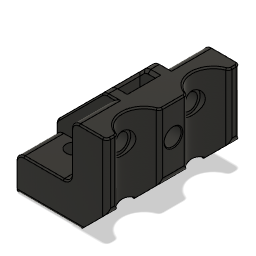
Apollo Yoke Int. Corner P2 [(P)MPLA000000157] v1 (Autodesk Fusion 360 design; units mm, degrees)
Autodesk Fusion 360 part; units mm, degrees
note: some values were not read from the file. Chosen so that the rebuilt part matches the saved one: which face or edge a step refers to; which pieces of a blend or face edit are solid. Set by a fixed rule: which sketch regions a step uses.
sketch "Sketch1" plane through (0, 0, 0) normal (0, 1, 0) x (1, 0, 0)
  line L0 (-17, 25) -> (-17, -25)
  line L1 (17, 25) -> (17, -25)
  line L2 (-17, -25) -> (17, -25)
  circle A0 centre (-19, 13) radius 8.1
  circle A1 centre (-19, -13) radius 8.1
  line L3 (-17, 25) -> (17, 25)
  circle A2 centre (19, 13) radius 8.1
  circle A3 centre (19, -13) radius 8.1
  dimension "d7" = 50
  dimension "d8" = 25
  dimension "d74" = 16.2
  dimension "d75" = 16.2
  dimension "d97" = 34
  dimension "d100" = 17
  dimension "d101" = 16.2
  dimension "d102" = 16.2
  dimension "d103" = 38
  dimension "d104" = 26
  dimension "d105" = 13
  dimension "d106" = 19
  constraint vertical L0
  constraint vertical L1
  constraint horizontal L2
  constraint horizontal L3
  constraint vertical A3.centre A2.centre
  constraint horizontal A0.centre A2.centre
  constraint horizontal A1.centre A3.centre
  constraint vertical A0.centre A1.centre
  measures "d7" distance of L2 L3
  measures "d8" distance of origin L2
  measures "d74" diameter of A3
  measures "d75" diameter of A2
  measures "d97" distance of L0 L1
  measures "d100" distance of origin L1
  measures "d101" diameter of A0
  measures "d102" diameter of A1
  measures "d103" distance of A0.centre A2.centre
  measures "d104" distance of A0.centre A1.centre
  measures "d105" vertical distance of origin A0.centre
  measures "d106" horizontal distance of origin A0.centre
extrude "Extrude1" add sketch "Sketch1" along normal blind 34 contours L0 L1 L2 A0 A1 L3 A2 A3 | L0 A0 | L0 A1 picked at (-15.419, 11.504) picked at (-14.0304, -14.3154)
sketch "Sketch3" plane through (17, 0, 0) normal (1, 0, 0) x (0, 0, -1)
  line L0 (20.8492, 0) -> (25, 0)
  line L1 (25, 0) -> (25, 34)
  line L2 (25, 34) -> (20.8492, 34)
  line L3 (-25, 34) -> (-25, 0)
  circle A0 centre (-13, -2) radius 8
  circle A1 centre (13, -2) radius 8.2
  circle A2 centre (-13, -2) radius 8.2
  circle A3 centre (13, -2) radius 8
  line L4 (20.8492, 34) -> (20.8492, 0)
  line L5 (-25, 0) -> (-20.8492, 0)
  line L6 (-20.8492, 0) -> (-20.8492, 34)
  line L7 (-20.8492, 34) -> (-25, 34)
  dimension "d34" = 0.2
  dimension "d35" = 0.2
  dimension "d36" = 16
  dimension "d37" = 16
  dimension "d38" = 26
  dimension "d39" = 13
  dimension "d40" = 2
  constraint concentric A0 A2
  constraint concentric A1 A3
  constraint horizontal A0.centre A1.centre
  measures "d36" diameter of A0
  measures "d37" diameter of A3
  measures "d38" distance of A0.centre A1.centre
  measures "d39" horizontal distance of origin A0.centre
  measures "d40" vertical distance of origin A0.centre
extrude "Extrude4" cut sketch "Sketch3" against normal blind 34 contours A0 | A3
chamfer "Chamfer4" distance 10 angle 45 7 edges at (17, 0, -22.9246) (17, 0, 22.9246) (17, 0, -22.9246) (17, 0, 0) (17, 0, 22.9246) (17, 0, 0) (17, 0, -22.9246)
chamfer "Chamfer5" distance 18 angle 45 1 edges at (-17, 34, 0)
fillet "Fillet3" radius 1.5 12 edges at (-5, 0, -25) (-5, 0, 25) (-5, 0, 5.254) (-5, 0, 20.746) (-5, 0, -5.254) (-5, 0, -20.746) (17, 22, 20.8492) (17, 22, 5.1508) (17, 22, -5.1508) (17, 22, -20.8492) (17, 22, -25) (17, 22, 25)
fillet "Fillet4" radius 3 8 edges at (7, 0, -22.6659) (17, 10, -22.7196) (17, 10, 0) (7, 0, 0) (7, 0, 22.6659) (17, 10, 22.7196) (-17, 16, 0) (1, 34, 0)
chamfer "Chamfer3" distance 0.5 angle 45 41 edges at (8.8713, 34, -25) (1.0946, 33.7716, -25) (-8, 25, -25) (-16.7716, 15.9054, -25) (-17, 8.1287, -25) (-17, 0.4393, -24.5607) (-17, 0, -22.6659) (-17, 0.2592, -20.9888) (-17, 6, -13) (-17, 0.2592, -5.0112) (-17, 0, 0) (-17, 0, 22.6659) (-17, 0, -22.6659) (-17, 0.2592, 20.9888) (-17, 0.2592, 5.0112) (-17, 6, 13) (-17, 0.2592, 20.9888) (-17, 0, 22.6659) (-17, 0.4393, 24.5607) (-17, 8.1287, 25) (-16.7716, 15.9054, 25) (-8, 25, 25) (1.0946, 33.7716, 25) (8.8713, 34, 25) (16.5607, 34, 24.5607) (17, 34, 22.7196) (16.739, 34, 21.0938) (10.9, 34, 13) (16.739, 34, 21.0938) (16.739, 34, 4.9062) (17, 34, -22.7196) (17, 34, 22.7196) (17, 34, 0) (16.739, 34, -4.9062) (10.9, 34, -13) (16.739, 34, -4.9062) (16.739, 34, -21.0938) (17, 34, 0) (17, 34, -22.7196) (17, 34, 22.7196) (16.5607, 34, -24.5607)
sketch "Sketch2" plane through (17, 0, 0) normal (1, 0, 0) x (0, 0, -1)
  circle A0 centre (0, 22.5) radius 3.1
  circle A1 centre (0, 22.5) radius 5.5
  line L0 (4.0608, 33.5) -> (-4.0608, 33.5)
  line L1 (-4.0608, 33.5) -> (-4.0608, 11.2426)
  line L2 (-4.0608, 11.2426) -> (4.0608, 11.2426)
  line L3 (4.0608, 11.2426) -> (4.0608, 33.5)
  line L4 (-4.9919, 34) -> (-21.0081, 34)
  dimension "d15" = 6.2
  dimension "d17" = 11
  dimension "d107" = 11.5
  constraint vertical origin A0.centre
  constraint concentric A0 A1
  measures "d15" diameter of A0
  measures "d17" diameter of A1
  measures "d107" distance of A0.centre L4
hole "Hole1" at (17, 22.5, 0) direction (-1, 0, 0) diameter 6.4 depth 21 tip angle 118 countersink diameter 7 countersink angle 90
sketch "Sketch4" plane through (0, 0, 0) normal (0, -1, 0) x (1, 0, 0)
  circle A0 centre (-5.5, 0) radius 3
  line L0 (-5.5, 4.1682) -> (-5.5, -4.1682)
  line L1 (5.259, -23.5) -> (5.259, -21.8318)
  line L2 (5.259, -21.8318) -> (-5.259, -21.8318)
  line L3 (-5.259, -21.8318) -> (-5.259, -23.5)
  line L4 (-5.259, -23.5) -> (5.259, -23.5)
  line L5 (5.7574, -4.1682) -> (5.7574, 4.1682)
  line L6 (5.7574, 4.1682) -> (-16.5, 4.1682)
  line L7 (-16.5, -4.1682) -> (5.7574, -4.1682)
  line L8 (-16.5, 4.1682) -> (-16.5, -4.1682)
  line L9 (-17, 4.1682) -> (-17, -4.1682)
  dimension "d66" = 6
  dimension "d110" = 11.5
  constraint horizontal origin A0.centre
  constraint midpoint A0.centre L0
  measures "d66" diameter of A0
  measures "d110" distance of A0.centre L9
hole "Hole2" at (-5.5, 0, 0) direction (0, 1, 0) diameter 6.4 depth 21 tip angle 118 countersink diameter 7 countersink angle 90
sketch "Sketch6" plane through (0, 34, 0) normal (0, 1, 0) x (-1, 0, 0)
  line L0 (-2.2426, 24.5) -> (-15.5, 24.5)
  arc A0 (-15.5, 24.5) -> (-16.5, 23.5) centre (-15.5, 23.5) ccw
  line L1 (-16.5, 23.5) -> (-16.5, 21.9392)
  arc A1 (-16.5, 21.9392) -> (-15.8646, 21.0081) centre (-15.5, 21.9392) ccw
  arc A2 (-15.8646, 4.9919) -> (-15.8646, 21.0081) centre (-19, 13) ccw
  arc A3 (-15.8646, 4.9919) -> (-16.5, 4.0608) centre (-15.5, 4.0608) ccw
  line L2 (-16.5, 4.0608) -> (-16.5, -4.0608)
  arc A4 (-16.5, -4.0608) -> (-15.8646, -4.9919) centre (-15.5, -4.0608) ccw
  arc A5 (-15.8646, -21.0081) -> (-15.8646, -4.9919) centre (-19, -13) ccw
  arc A6 (-15.8646, -21.0081) -> (-16.5, -21.9392) centre (-15.5, -21.9392) ccw
  line L3 (-16.5, -21.9392) -> (-16.5, -23.5)
  arc A7 (-16.5, -23.5) -> (-15.5, -24.5) centre (-15.5, -23.5) ccw
  line L4 (-15.5, -24.5) -> (-2.2426, -24.5)
  line L5 (-2.2426, -24.5) -> (-2.2426, 24.5)
  line L6 (-17, 4.0608) -> (-17, -4.0608)
  line L7 (-5, -5.25) -> (0.8, -5.25)
  line L8 (0.8, -5.25) -> (0.8, 5.25)
  line L9 (0.8, 5.25) -> (-5, 5.25)
  line L10 (-5, 5.25) -> (-5, -5.25)
  line L11 (-5, -5.25) -> (0.8, 5.25) construction
  line L12 (0.8, -5.25) -> (-5, 5.25) construction
  point P0 (-2.1, 0)
  dimension "d144" = 5.8
  dimension "d145" = 10.5
  dimension "d146" = 5.25
  dimension "d149" = 12
  constraint horizontal L7
  constraint perpendicular L7 L8
  constraint parallel L7 L9
  constraint parallel L8 L10
  constraint coincident L11 P0
  constraint coincident L12 P0
  measures "d144" distance of L8 L10
  measures "d145" distance of L7 L9
  measures "d146" distance of origin L7
  measures "d149" distance of L6 L10
extrude "Extrude5" cut sketch "Sketch6" against normal blind 13 contours L5 L7 L8 L9 | L5 L7 L9 L10
sketch "Sketch8" plane through (5, 0, 0) normal (-1, 0, 0) x (0, 0, 1)
  arc A0 (2.8267, 21) -> (-2.8267, 21) centre (0, 22.5) ccw
  line L0 (2.8267, 21) -> (5.25, 21)
  line L1 (5.25, 21) -> (5.25, 34)
  line L2 (5.25, 34) -> (-5.25, 34)
  line L3 (-5.25, 34) -> (-5.25, 21)
  line L4 (-5.25, 21) -> (-2.8267, 21)
  line L5 (5.25, 25.0311) -> (0, 28.0622)
  line L6 (0, 28.0622) -> (-5.25, 25.0311)
  line L7 (-5.25, 25.0311) -> (-5.25, 18.9689)
  line L8 (-5.25, 18.9689) -> (0, 15.9378)
  line L9 (0, 15.9378) -> (5.25, 18.9689)
  line L10 (5.25, 18.9689) -> (5.25, 25.0311)
  point P0 (0, 22)
  dimension "d156" = 0.5
  constraint collinear L3 L7
  constraint vertical A0.centre P0
  measures "d156" distance of A0.centre P0
extrude "Extrude7" cut sketch "Sketch8" along normal up to surface (5.8 mm away) contours A0 L0 L4 L7 L8 L9 L10
sketch "Sketch7" plane through (-17, 0, 0) normal (-1, 0, 0) x (0, 0, 1)
  line L0 (24.5, 1.5) -> (24.5, 14.7574)
  line L1 (24.5, 14.7574) -> (-24.5, 14.7574)
  line L2 (-24.5, 14.7574) -> (-24.5, 1.5)
  arc A0 (-24.5, 1.5) -> (-23.5, 0.5) centre (-23.5, 1.5) ccw
  line L3 (-23.5, 0.5) -> (-21.8318, 0.5)
  arc A1 (-21.8318, 0.5) -> (-20.9021, 1.1316) centre (-21.8318, 1.5) ccw
  arc A2 (-5.0979, 1.1316) -> (-20.9021, 1.1316) centre (-13, -2) ccw
  arc A3 (-5.0979, 1.1316) -> (-4.1682, 0.5) centre (-4.1682, 1.5) ccw
  line L4 (-4.1682, 0.5) -> (4.1682, 0.5)
  arc A4 (4.1682, 0.5) -> (5.0979, 1.1316) centre (4.1682, 1.5) ccw
  arc A5 (20.9021, 1.1316) -> (5.0979, 1.1316) centre (13, -2) ccw
  arc A6 (20.9021, 1.1316) -> (21.8318, 0.5) centre (21.8318, 1.5) ccw
  line L5 (21.8318, 0.5) -> (23.5, 0.5)
  arc A7 (23.5, 0.5) -> (24.5, 1.5) centre (23.5, 1.5) ccw
  line L6 (-4.1682, 0) -> (4.1682, 0)
  line L7 (5.25, 17.8) -> (-5.25, 17.8)
  line L8 (-5.25, 17.8) -> (-5.25, 12)
  line L9 (-5.25, 12) -> (5.25, 12)
  line L10 (5.25, 12) -> (5.25, 17.8)
  line L11 (5.25, 17.8) -> (-5.25, 12) construction
  line L12 (-5.25, 17.8) -> (5.25, 12) construction
  line L13 (-5.25, 32.2) -> (-5.25, 33.1213)
  point P0 (0, 14.9)
  dimension "d128" = 10.5
  dimension "d129" = 5.8
  dimension "d148" = 12
  constraint horizontal L7
  constraint perpendicular L7 L8
  constraint parallel L7 L9
  constraint parallel L8 L10
  constraint coincident L11 P0
  constraint coincident L12 P0
  constraint collinear L8 L13
  measures "d128" distance of L8.end L9.end
  measures "d129" distance of L7.end L8.end
  measures "d148" distance of origin L9
extrude "Extrude6" cut sketch "Sketch7" against normal blind 13 contours L1 L8 L9 L10 | L1 L7 L8 L10
sketch "Sketch9" plane through (0, 12, 0) normal (0, 1, 0) x (-1, 0, 0)
  line L0 (4, -2.8267) -> (4, -5.25)
  line L1 (4, -5.25) -> (17, -5.25)
  line L2 (17, -5.25) -> (17, 5.25)
  line L3 (17, 5.25) -> (4, 5.25)
  line L4 (4, 5.25) -> (4, 2.8267)
  arc A0 (4, -2.8267) -> (4, 2.8267) centre (5.5, 0) ccw
  line L5 (8.0311, -5.25) -> (11.0622, 0)
  line L6 (11.0622, 0) -> (8.0311, 5.25)
  line L7 (8.0311, 5.25) -> (1.9689, 5.25)
  line L8 (1.9689, 5.25) -> (-1.0622, 0)
  line L9 (-1.0622, 0) -> (1.9689, -5.25)
  line L10 (1.9689, -5.25) -> (8.0311, -5.25)
  point P0 (5.5, 0)
  point P1 (5.5, 0)
  point P2 (5, 0)
  dimension "d157" = 0.5
  constraint coincident P1 P0
  constraint collinear L1 L10
  constraint horizontal P1 P2
  measures "d157" distance of P1 P2
extrude "Extrude8" cut sketch "Sketch9" along normal up to surface (5.8 mm away) contours L0 L1 L3 L4 A0 L5 L6 L7 L10 | L0 L4 A0 L7 L8 L9 L10
chamfer "Chamfer8" distance 2 angle 45 1 edges at (-0.8, 17.8, 0)
chamfer "Chamfer6" distance 1 angle 45 14 edges at (-16.7716, 15.9054, 5.25) (-15.6607, 17.3393, 5.25) (-17, 13.3787, 5.25) (-16.7716, 15.9054, -5.25) (-17, 13.3787, -5.25) (-15.6607, 17.3393, -5.25) (3.6213, 34, 5.25) (1.0946, 33.7716, 5.25) (-0.3393, 32.6607, 5.25) (3.6213, 34, -5.25) (1.0946, 33.7716, -5.25) (-0.3393, 32.6607, -5.25) (5, 34, 0) (-17, 12, 0)
sketch "Sketch10" plane through (0, 0, 25) normal (0, 0, 1) x (1, 0, 0)
  line L0 (-16.5, 14.7574) -> (-16.5, 1.5)
  line L1 (-16.5, 1.5) -> (8.5, 1.5)
  line L2 (8.5, 1.5) -> (15.5, 8.5)
  line L3 (15.5, 8.5) -> (15.5, 33.5)
  line L4 (15.5, 33.5) -> (2.2426, 33.5)
  arc A0 (2.2426, 33.5) -> (0.4749, 32.7678) centre (2.2426, 31) ccw
  line L5 (0.4749, 32.7678) -> (-15.7678, 16.5251)
  arc A1 (-15.7678, 16.5251) -> (-16.5, 14.7574) centre (-14, 14.7574) ccw
  line L6 (3.7426, 13.2574) -> (-20.6124, 13.2574)
  line L7 (-20.6124, 13.2574) -> (-3.4252, 34.9761)
  line L8 (-3.4252, 34.9761) -> (3.7426, 34.9761)
  line L9 (3.7426, 13.2574) -> (3.7426, 34.9761)
  dimension "d134" = 1.5
  dimension "d135" = 1.5
  constraint perpendicular L0 L6
  constraint horizontal L8
  constraint vertical L9
  measures "d134" distance of L4.end L9
  measures "d135" distance of L0.start L6
extrude "Extrude9" cut sketch "Sketch10" against normal blind 15 contours L0 L4 A0 L5 A1 L6 L9 | L0 L4 A0 L5 A1 L6 L7 L8 L9
extrude "Extrude10" cut sketch "Sketch10" along normal blind 15 from surface at -50 contours L0 L4 A0 L5 A1 L6 L9 | L0 L4 A0 L5 A1 L6 L7 L8 L9
fillet "Fillet5" radius 3 6 edges at (3.7426, 34, 17.25) (-17, 13.2574, 17.25) (3.7426, 13.2574, 17.5) (-17, 13.2574, -17.25) (3.7426, 13.2574, -17.5) (3.7426, 34, -17.25)
chamfer "Chamfer7" distance 0.5 angle 45 20 edges at (3.7426, 23.6287, 25) (2.864, 14.136, 25) (-6.6287, 13.2574, 25) (-15.4186, 12.9007, 25) (4.0993, 32.4186, 25) (3.7426, 23.6287, -25) (4.0993, 32.4186, -25) (-15.4186, 12.9007, -25) (-6.6287, 13.2574, -25) (2.864, 14.136, -25) (-8, 25, -10) (-16.7716, 15.9054, -10) (-17, 12.5074, -10) (4.4926, 34, -10) (1.0946, 33.7716, -10) (-8, 25, 10) (1.0946, 33.7716, 10) (4.4926, 34, 10) (-17, 12.5074, 10) (-16.7716, 15.9054, 10)
chamfer "Chamfer10" distance 1.4 angle 45 2 edges at (-0.8, 32.2, 0) (-15.2, 17.8, 0)
sketch "Sketch11" plane through (0, 0, -5.25) normal (0, 0, 1) x (1, 0, 0)
  line L0 (-0.8, 19.8) -> (-1.6311, 18.9689)
  line L1 (-0.8, 25.6966) -> (-8.6966, 17.8)
  line L2 (-8.6966, 16.4221) -> (-2.5708, 16.4221)
  line L3 (-2.5708, 16.4221) -> (0.213, 19.206)
  line L4 (0.213, 19.206) -> (0.213, 25.6966)
  line L5 (0.213, 25.6966) -> (-0.8, 25.6966)
  line L6 (-8.6966, 17.8) -> (-8.6966, 16.4221)
  line L7 (-13.7858, 17.8) -> (-15.4142, 16.1716)
  arc A0 (-15.4142, 16.1716) -> (-16, 14.7574) centre (-14, 14.7574) ccw
  line L8 (-16, 14.7574) -> (-16, 12)
  line L9 (-16, 12) -> (-1.9689, 12)
  line L10 (-2.8, 17.8) -> (-13.7858, 17.8)
  line L11 (5.1492, 19.0162) -> (-1.9689, 12)
  line L12 (5.1492, 19.0162) -> (-0.8, 19.8)
  line L13 (-1.9689, 12) -> (-1.6311, 18.9689)
  line L14 (5, 33) -> (2.2426, 33)
  arc A1 (2.2426, 33) -> (0.8284, 32.4142) centre (2.2426, 31) ccw
  line L15 (0.8284, 32.4142) -> (-0.8, 30.7858)
  line L16 (-0.8, 30.7858) -> (-0.8, 19.8)
  line L17 (-1.6311, 18.9689) -> (5, 18.9689)
  line L18 (5, 18.9689) -> (5, 33)
  line L19 (-1.9689, 12) -> (-1.9689, 18.6311)
  line L20 (-1.9689, 18.6311) -> (-2.8, 17.8)
  point P0 (-0.8, 19.8)
  point P1 (5, 18.9689)
  point P2 (-0.8, 30.7858)
  point P3 (5, 33)
  point P4 (-0.8, 19.8)
  constraint parallel L1 L3
  constraint parallel L0 L3
  constraint perpendicular L2 L6
  constraint coincident L9.end L11.end
  constraint coincident P4 P0
  constraint coincident L0.end L13.end
extrude "Extrude11" cut sketch "Sketch11" along normal up to surface (10.5 mm away) contours L0 L3 L4 L12 L17 | L0 L1 L3 L10 L13 L16 L19 L20 | L3 L13 L17 | L3 L4 L12 L17 L18 | L2 L3 L6 L10 L19 L20
sketch "Sketch12" plane through (17, 0, 0) normal (1, 0, 0) x (0, 0, -1)
  circle A0 centre (0, 22.5) radius 3.5
  line L0 (4.0608, 33.5) -> (-4.0608, 33.5)
  line L1 (-4.0608, 33.5) -> (-4.0608, 11.2426)
  line L2 (-4.0608, 11.2426) -> (4.0608, 11.2426)
  line L3 (4.0608, 11.2426) -> (4.0608, 33.5)
  circle A1 centre (-13, 24) radius 3
  circle A2 centre (13, 24) radius 3
  line L4 (4.0608, 34) -> (-4.0608, 34)
  arc A3 (-5.5627, 0.9474) -> (-20.4373, 0.9474) centre (-13, -2) ccw
  circle A4 centre (13, 24) radius 4
  circle A5 centre (-13, 24) radius 4
  dimension "d159" = 6
  dimension "d161" = 6
  dimension "d164" = 26
  dimension "d165" = 13
  dimension "d181" = 18
  dimension "d185" = 8
  dimension "d186" = 8
  constraint horizontal A1.centre A2.centre
  constraint concentric A2 A4
  constraint concentric A1 A5
  measures "d159" diameter of A1
  measures "d161" diameter of A2
  measures "d164" distance of A1.centre A2.centre
  measures "d165" horizontal distance of origin A1.centre
  measures "d181" distance of A1.centre A3
  measures "d185" diameter of A4
  measures "d186" diameter of A5
extrude "Extrude16" cut sketch "Sketch12" against normal blind 30 contours A1 | A2
extrude "Extrude17" cut sketch "Sketch12" against normal blind 7 contours A4 | A5
sketch "Sketch13" plane through (0, 0, 0) normal (0, -1, 0) x (1, 0, 0)
  circle A0 centre (-5.5, 0) radius 3.5
  line L0 (-16.5, 4.1682) -> (-16.5, -4.1682)
  line L1 (-16.5, -4.1682) -> (5.7574, -4.1682)
  line L2 (5.7574, -4.1682) -> (5.7574, 4.1682)
  line L3 (5.7574, 4.1682) -> (-16.5, 4.1682)
  circle A1 centre (-7.1, 13) radius 3
  circle A2 centre (-7.1, -13) radius 3
  line L4 (-17, 4.1682) -> (-17, -4.1682)
  arc A3 (16.0469, -5.4575) -> (16.0469, -20.5425) centre (19, -13) ccw
  circle A4 centre (-7.1, 13) radius 4
  circle A5 centre (-7.1, -13) radius 4
  dimension "d172" = 6
  dimension "d173" = 6
  dimension "d174" = 26
  dimension "d175" = 13
  dimension "d182" = 18
  dimension "d189" = 8
  dimension "d190" = 8
  constraint vertical A1.centre A2.centre
  constraint concentric A1 A4
  constraint concentric A2 A5
  measures "d172" diameter of A1
  measures "d173" diameter of A2
  measures "d174" distance of A1.centre A2.centre
  measures "d175" vertical distance of origin A1.centre
  measures "d182" distance of A2.centre A3
  measures "d189" diameter of A4
  measures "d190" diameter of A5
extrude "Extrude14" cut sketch "Sketch13" against normal blind 15 contours A1 | A2
extrude "Extrude15" cut sketch "Sketch13" against normal blind 7 contours A1 | A4 | A5
equation "d8 = d7 / 2"
equation "d39 = d38 / 2"
equation "d100 = d97 / 2"
equation "d105 = d104 / 2"
equation "d106 = d103 / 2"
equation "d146 = d145 / 2"
equation "d165 = d164 / 2"
equation "d175 = d174 / 2"
